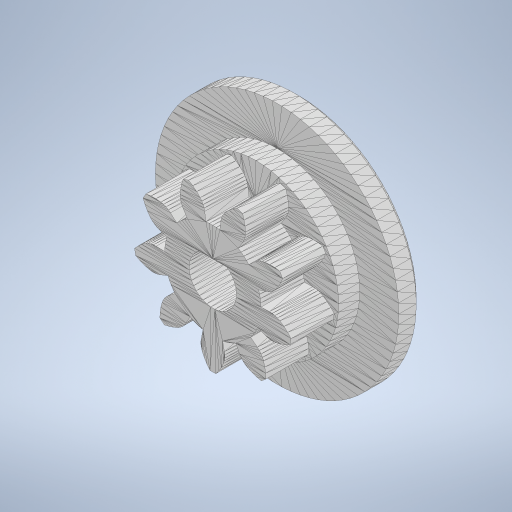
# Autodesk Inventor part: 06-Gear
Saved by Autodesk Inventor 2023.2 (Build 272271000, 271)
## iProperties
Created: 2023-03-17
Part Number: 06-Gear
Material: Generisch
Document SubType Name: Modeling
Designer: hangel
Density: 1 g/cm^3
Appearance: Vorgabe
Author: hangel
Autodesk Inventor part; units mm, degrees
ref_plane "YZ Plane" through (0, 0, 0) normal (1, 0, 0) x (0, 1, 0)
ref_plane "XZ Plane" through (0, 0, 0) normal (0, 1, 0) x (-1, 0, 0)
ref_plane "XY Plane" through (0, 0, 0) normal (0, 0, 1) x (1, 0, 0)
sketch "Skizze2" plane through (0, -12.75, 0) normal (0, 0, -1) x (-1, 0, 0)
  circle A0 centre (0, 12.75) radius 3.5749 projected
  line L0 (-1.5248, 14.825) -> (1.5248, 14.825) projected
  point P0 (0, 12.75)
sketch "Skizze3" plane through (0.8023, 2.4468, 5.5) normal (0, 0, -1) x (-1, 0, 0)
  circle A0 centre (0.8023, -2.4468) radius 2.575 projected
  line L0 (-0.7225, -0.3718) -> (2.3271, -0.3718) projected
  point P0 (0.8023, -2.4468)
extrude "Extrusion2" add sketch "Skizze3" along normal blind 3.5 contours L0 A0 picked at (1.1542, -0.2806)
chamfer "Fase2" distance 0.45 angle 45 1 edges at (0, 2.075, 2)
